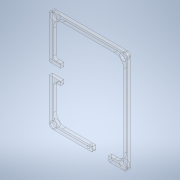
# Autodesk Inventor part: Plex_Rand_untere2
Saved by Autodesk Inventor 2022 (Build 260153000, 153)
## iProperties
Created: 2021-06-16
Part Number: Plex_Rand_untere2
Material: PET Plastic
Document SubType Name: Modeling
Designer: domin
Density: 1.541 g/cm^3
Appearance: Polycarbonate - Clear
Mass: 28.0983 g
Surface Area: 135.189 cm^2
Volume: 18.2338 cm^3
Author: domin
Autodesk Inventor part; units mm, degrees
ref_plane "YZ Plane" through (0, 0, 0) normal (1, 0, 0) x (0, 1, 0)
ref_plane "XZ Plane" through (0, 0, 0) normal (0, 1, 0) x (-1, 0, 0)
ref_plane "XY Plane" through (0, 0, 0) normal (0, 0, 1) x (1, 0, 0)
sketch "Sketch1" plane through (0, 0, 0) normal (0, 0, 1) x (1, 0, 0)
  line L0 (-57, -81) -> (7, -81)
  line L1 (62, -76) -> (62, -22)
  line L2 (57, 81) -> (-57, 81)
  line L3 (-62, 76) -> (-62, 9)
  line L4 (-41, -73) -> (7, -73)
  line L5 (56, -58) -> (56, -22)
  line L6 (41, 73) -> (-41, 73)
  line L7 (-56, 58) -> (-56, 20)
  arc A0 (-56, -58) -> (-41, -73) centre (-41, -58) ccw
  arc A1 (-41, 73) -> (-56, 58) centre (-41, 58) ccw
  arc A2 (56, 58) -> (41, 73) centre (41, 58) ccw
  arc A3 (41, -73) -> (56, -58) centre (41, -58) ccw
  line L8 (56, -22) -> (62, -22) construction
  line L9 (56, -10) -> (62, -10) construction
  line L10 (-56, 9) -> (-62, 9)
  line L11 (-62, -22) -> (-56, -22) construction
  line L12 (-62, -22) -> (-62, -76)
  line L13 (-62, 9) -> (-62, -9) construction
  line L14 (-56, -22) -> (-56, -58)
  line L15 (56, -22) -> (56, -10)
  line L16 (56, -10) -> (56, 58)
  line L17 (62, -22) -> (62, -10)
  line L18 (62, -10) -> (62, 76)
  arc A4 (-62, -76) -> (-57, -81) centre (-57, -76) ccw
  arc A5 (-57, 81) -> (-62, 76) centre (-57, 76) ccw
  arc A6 (62, 76) -> (57, 81) centre (57, 76) ccw
  arc A7 (57, -81) -> (62, -76) centre (57, -76) ccw
  circle A8 centre (-55, -74) radius 5.25
  line L19 (-92.4325, 0) -> (79.0499, 0) construction
  line L20 (0, -100.3717) -> (0, 120.689) construction
  circle A9 centre (-55, 74) radius 5.25
  circle A10 centre (55, -74) radius 5.25
  circle A11 centre (55, 74) radius 5.25
  line L21 (-64, -9) -> (-62, -9)
  line L22 (-62, -9) -> (-62, -22)
  line L23 (-64, -9) -> (-44, -9)
  line L24 (-44, 9) -> (-56, 9)
  line L25 (-51, 15) -> (-44, 15)
  line L26 (-44, 15) -> (-44, 9)
  line L27 (-44, -15) -> (-51, -15)
  line L28 (-44, -9) -> (-44, -15)
  line L29 (-56, -20) -> (-56, -22)
  arc A12 (-56, 20) -> (-51, 15) centre (-51, 20) ccw
  arc A13 (-51, -15) -> (-56, -20) centre (-51, -20) ccw
  line L30 (7, -81) -> (7, -73)
  line L31 (32, -81) -> (32, -73)
  line L32 (7, -81) -> (32, -81) construction
  line L33 (7, -73) -> (32, -73) construction
  line L34 (32, -73) -> (41, -73)
  line L35 (32, -81) -> (57, -81)
  circle A14 centre (0, -77) radius 2.1
  point P0 (0, 0)
  point P1 (-62, -81)
  point P2 (62, 81)
  point P3 (-62, 81)
  point P4 (-44, -12)
  point P5 (-59, 9)
  dimension "d0" = 162
  dimension "d1" = 124
  dimension "d2" = 62
  dimension "d3" = 81
  dimension "d4" = 6
  dimension "d5" = 8
  dimension "d6" = 6
  dimension "d7" = 8
  dimension "d8" = 15
  dimension "d9" = 12
  dimension "d10" = 59
  dimension "d11" = 59
  dimension "d12" = 72
  dimension "d13" = 5
  dimension "d14" = 7
  dimension "d15" = 7
  dimension "d16" = 10.5
  dimension "d19" = 72
  dimension "d21" = 12
  dimension "d22" = 6
  dimension "d23" = 6
  dimension "d24" = 5
  dimension "d25" = 25
  dimension "d26" = 30
  dimension "d27" = 4.2
  dimension "d28" = 4
  constraints: 72 end point, 41 perpendicular, 36 tangent, 29 parallel, 20 point on circle, 15 centre point, 15 point on line, 9 horizontal, 7 equal radius, 3 symmetric about line, 2 midpoint, 1 vertical, 3 other
  measures "d0" distance of point (-62, 81) point (-62, -81)
  measures "d1" distance of point (62, 81) point (-62, 81)
  measures "d2" distance from line of L3 point (0, 0)
  measures "d3" distance from line of point (0, 0) L0
  measures "d4" distance between parallel lines of L3 L7
  measures "d5" distance between parallel lines of L0 L4
  measures "d6" distance between parallel lines of L1 L5
  measures "d7" distance between parallel lines of L2 L6
  measures "d8" radius of A0
  measures "d9" distance between parallel lines of L9 L8
  measures "d10" distance between parallel lines of L8 L0
  measures "d11" distance between parallel lines of L0 L11
  measures "d12" distance between parallel lines of L2 L10
  measures "d13" radius of A4
  measures "d14" distance from line of A8.centre L12
  measures "d15" distance from line of A8.centre L0
  measures "d16" diameter of A8
  measures "d19" distance between parallel lines of L0 L21
  measures "d21" distance between parallel lines of L14 L28
  measures "d22" distance between parallel lines of L27 L23
  measures "d23" distance between parallel lines of L24 L25
  measures "d24" radius of A12
  measures "d25" distance between parallel lines of L31 L30
  measures "d26" distance between parallel lines of L31 L1
  measures "d27" diameter of A14
  measures "d28" distance from line of L0 A14.centre
extrude "Extrusion1" add sketch "Sketch1" along normal blind 5
fillet "Fillet1" radius 2 3 edges at (-62, 9, 2.5) (7, -81, 2.5) (32, -81, 2.5)
equation "\"d23\" = d22"
body "Solid1"
